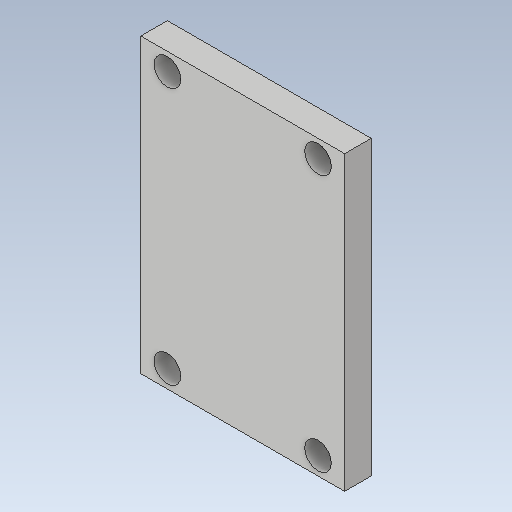
# Autodesk Inventor part: case_core
Saved by Autodesk Inventor 2020.1 (Build 241239000, 239)
## iProperties
Created: 2018-05-21
Part Number: case_core
Material: Generic
Document SubType Name: Modeling
Designer: Bardo91
Density: 1 g/cm^3
Appearance: Default
Author: Bardo91
Autodesk Inventor part; units mm, degrees
ref_plane "YZ Plane" through (0, 0, 0) normal (1, 0, 0) x (0, 1, 0)
ref_plane "XZ Plane" through (0, 0, 0) normal (0, 1, 0) x (-1, 0, 0)
ref_plane "XY Plane" through (0, 0, 0) normal (0, 0, 1) x (1, 0, 0)
sketch "Sketch1" plane through (0, 0, 0) normal (0, 0, 1) x (1, 0, 0)
  line L0 (0, 0) -> (23, 0)
  line L1 (23, 0) -> (23, 33)
  line L2 (23, 33) -> (0, 33)
  line L3 (0, 33) -> (0, 0)
  dimension "d0" = 23
  dimension "d1" = 33
  constraints: 8 end point, 2 parallel, 1 horizontal, 1 perpendicular
  measures "d0" distance of L2.end L1.end
  measures "d1" distance of L0.end L1.end
extrude "Extrusion1" add sketch "Sketch1" along normal blind 3
sketch "Sketch2" plane through (0, 0, 3) normal (0, 0, 1) x (1, 0, 0)
  line L0 (0, 0) -> (23, 0) projected
  line L1 (0, 0) -> (3, 0)
  line L2 (3, 0) -> (3, 2)
  circle A0 centre (3, 2) radius 1.5
  line L3 (23, 0) -> (20, 0)
  line L4 (20, 0) -> (20, 2)
  line L5 (23, 0) -> (23, 33) projected
  line L6 (23, 33) -> (20, 33)
  line L7 (20, 33) -> (20, 31)
  line L8 (0, 33) -> (3, 33)
  line L9 (23, 33) -> (0, 33) projected
  line L10 (3, 33) -> (3, 31)
  circle A1 centre (3, 31) radius 1.5
  circle A2 centre (20, 31) radius 1.5
  circle A3 centre (20, 2) radius 1.5
  dimension "d4" = 3
  dimension "d5" = 2
  dimension "d6" = 3
  dimension "d7" = 3
  dimension "d8" = 2
  dimension "d9" = 3
  dimension "d10" = 2
  dimension "d11" = 3
  dimension "d12" = 2
  dimension "d13" = 3
  dimension "d14" = 3
  dimension "d15" = 3
  constraints: 16 end point, 4 centre point, 4 coincident, 4 perpendicular, 3 point on line, 1 horizontal
  measures "d4" distance of L0.start L1.end
  measures "d5" distance of L1.end L2.end
  measures "d6" diameter of A0
  measures "d7" distance of L0.end L3.end
  measures "d8" distance of L3.end L4.end
  measures "d9" distance of L5.end L6.end
  measures "d10" distance of L6.end L7.end
  measures "d11" distance of L8.start L8.end
  measures "d12" distance of L8.end L10.end
  measures "d13" diameter of A1
  measures "d14" diameter of A2
  measures "d15" diameter of A3
extrude "Extrusion2" cut sketch "Sketch2" against normal through all
body "Solid1"
